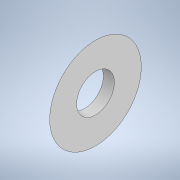
# Autodesk Inventor part: spacer2
Saved by Autodesk Inventor 2022 (Build 260153000, 153)
## iProperties
Created: 2022-02-18
Part Number: spacer2
Material: Genérico
Document SubType Name: Modeling
Designer: JK
Density: 1 g/cm^3
Appearance: Valor por defecto
Author: JK
Autodesk Inventor part; units mm, degrees
ref_plane "YZ Plane" through (0, 0, 0) normal (1, 0, 0) x (0, 1, 0)
ref_plane "XZ Plane" through (0, 0, 0) normal (0, 1, 0) x (-1, 0, 0)
ref_plane "XY Plane" through (0, 0, 0) normal (0, 0, 1) x (1, 0, 0)
sketch "Boceto1" plane through (0, 0, 0) normal (0, 1, 0) x (-1, 0, 0)
  line L0 (0, 0) -> (0, 2.25)
  line L1 (0, 2.25) -> (-0.96, 4)
  line L2 (-0.96, 4) -> (-0.96, 0)
  line L3 (-0.96, 0) -> (0, 0)
  line L4 (0, 1.65) -> (-0.96, 1.65)
  dimension "d0" = 1.65
  dimension "d1" = 2.25
  dimension "d2" = 0.96
  dimension "d3" = 4
  constraints: 10 end point, 2 perpendicular, 2 point on line, 1 parallel, 1 vertical
  measures "d0" distance between parallel lines of L3 L4
  measures "d1" distance of L0.start L0.end
  measures "d2" distance of L2.end L0.start
  measures "d3" distance of L1.end L2.end
revolve "Revolución1" add sketch "Boceto1" angle 360 about axis through (0.96, 0, 0) along (-1, 0, 0) contours L4 L2 L1 L0
